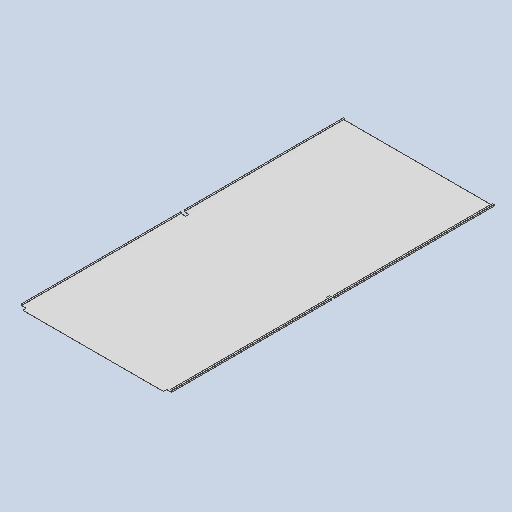
# Autodesk Inventor part: MSC 802 sheet gills
Saved by Autodesk Inventor 2025 (Build 290162010, 162A)
## iProperties
Created: 2024-06-15
Part Number: MSC 802 sheet gills
Material: Stainless Steel
Document SubType Name: Sheet Metal
Designer: pokla
Density: 8 g/cm^3
Sheet Metal Rule: Default_mm
Appearance: Default
Stock Number: МОО 802 лист жабра
Mass: 7522.03 g
Surface Area: 37640.3 cm^2
Volume: 940.254 cm^3
Flat Pattern Width: 95.1524 cm
Flat Pattern Length: 198 cm
Flat Pattern Area: 18840.2 cm^2
Sheet Metal Width: 951,524 mm
Sheet Metal Length: 1980,000 mm
Sheet Metal Area: 1884017,309 mm^2
Author: pokla
Autodesk Inventor part; units mm, degrees
ref_plane "YZ Plane" through (0, 0, 0) normal (1, 0, 0) x (0, 1, 0)
ref_plane "XZ Plane" through (0, 0, 0) normal (0, 1, 0) x (-1, 0, 0)
ref_plane "XY Plane" through (0, 0, 0) normal (0, 0, 1) x (1, 0, 0)
sketch "Sketch6" plane through (0, 0, 0) normal (0, 1, 0) x (-1, 0, 0)
  line L0 (457.5, -990) -> (-457.5, -990)
  line L1 (-457.5, -990) -> (-457.5, 990)
  line L2 (-457.5, 990) -> (457.5, 990)
  line L3 (457.5, 990) -> (457.5, -990)
  line L4 (457.5, -990) -> (-457.5, 990) construction
  line L5 (-457.5, -990) -> (457.5, 990) construction
  point P0 (0, 0)
  dimension "d52" = 915
  dimension "d53" = 1980
  measures "d52" distance of L1.end L2.end
  measures "d53" distance of L0.end L1.end
extrude "Plate2" add sketch "Sketch6" along normal blind 0.5
sketch "Sketch10" plane through (-457, 0, 990) normal (-1, 0, 0) x (0, -1, 0)
  line L0 (0, -1980) -> (0, 0)
  line L1 (0, 0) -> (-10, 0)
  line L2 (-10, 0) -> (-10, -1980)
  line L3 (-10, -1980) -> (0, -1980)
  constraints: 6 end point, 1 horizontal, 1 perpendicular, 1 vertical
edge flange "Flange1" height 10 angle 90 thickness 0.5 bend radius 0.5 thickness toward (-1, 0, 0) relief straight relief width 0.5 relief depth 0.25 corner gap 0.5 corner form 0 edges at (-457.5, 0.5, 0) (457.5, 0.5, 0) wall of the first edge with corners at (-457, 0, -990) (-457, 0, 990) (-457, 10, 990) (-457, 10, -990)
bend "Bend2"
corner "Corner2"
sketch "Sketch11" plane through (457.5, 9.5, -990) normal (0, 1, 0) x (-1, 0, 0)
  line L0 (0, 1980) -> (0, 0)
  line L1 (0, 0) -> (10, 0)
  line L2 (10, 0) -> (10, 1980)
  line L3 (10, 1980) -> (0, 1980)
  constraints: 6 end point, 1 horizontal, 1 perpendicular, 1 vertical
edge flange "Flange2" height 10 angle 90 thickness 0.5 bend radius 0.5 thickness toward (0, 1, 0) relief straight relief width 0.5 relief depth 0.25 corner gap 0.5 corner form 0 edges at (457, 10, 0) (-457, 10, 0) wall of the first edge with corners at (457.5, 9.5, 990) (457.5, 9.5, -990) (447.5, 9.5, -990) (447.5, 9.5, 990)
bend "Bend3"
corner "Corner3"
sketch "Sketch12" plane through (0, 0, 0) normal (0, -1, 0) x (1, 0, 0)
  line L0 (457.5, -990) -> (457.5, 990) projected
  line L1 (457.5, 990) -> (457.5, -990) projected
  line L2 (-457.5, 990) -> (-427.5, 990)
  line L3 (-427.5, 990) -> (-427.5, 970)
  line L4 (-427.5, 970) -> (-457.5, 970)
  line L5 (-457.5, 970) -> (-457.5, 990)
  line L6 (-457.5, 0) -> (-427.5, 0)
  line L7 (-427.5, 0) -> (-427.5, -20)
  line L8 (-427.5, -20) -> (-457.5, -20)
  line L9 (-457.5, -20) -> (-457.5, 0)
  line L10 (457.5, 0) -> (427.5, 0)
  line L11 (427.5, 0) -> (427.5, -20)
  line L12 (427.5, -20) -> (457.5, -20)
  line L13 (457.5, -20) -> (457.5, 0)
  line L14 (456.5, -990) -> (456.5, 990) construction
  line L15 (457.5, 990) -> (427.5, 990)
  line L16 (427.5, 990) -> (427.5, 970)
  line L17 (427.5, 970) -> (457.5, 970)
  line L18 (457.5, 970) -> (457.5, 990)
  line L19 (-456.5, 990) -> (456.5, 990) projected
  line L20 (-457.5, -990) -> (-457.5, 990) projected
  point P0 (0, 0)
  point P1 (457.5, -20)
  point P2 (457.5, 0)
  point P3 (457.5, 970)
  dimension "d96" = 20
  dimension "d97" = 30
  dimension "d109" = 990
  dimension "d110" = 30
  constraints: 32 end point, 8 parallel, 4 collinear, 4 horizontal, 4 perpendicular, 3 equal length, 1 midpoint
  measures "d96" distance of L2.end L3.end
  measures "d97" distance of L2.start L2.end
  measures "d109" distance between parallel lines of L6 L2
  measures "d110" distance of L16.end L17.end
extrude "Extrusion3" cut sketch "Sketch12" against normal through all
fillet "Corner Round1" radius 4 16 edges at (-427.5, 0.25, 990) (-427.5, 0.25, 970) (-447.5, 9.75, 970) (427.5, 0.25, 990) (447.5, 9.75, 970) (427.5, 0.25, 970) (447.5, 9.75, 0) (447.5, 9.75, -20) (427.5, 0.25, -20) (427.5, 0.25, 0) (447.5, 9.75, -990) (-447.5, 9.75, -990) (-447.5, 9.75, 0) (-427.5, 0.25, 0) (-427.5, 0.25, -20) (-447.5, 9.75, -20)
equation "\"d52\" = ЖАБРЫ_базовая_ширина"
equation "\"d53\" = ЖАБРЫ_базовая_длина_дл_лист"
equation "\"d110\" = d97"
equation "\"d54\" = Thickness"
equation "\"d74\" = BendReliefWidth"
equation "\"d75\" = BendReliefDepth"
equation "\"d76\" = MinimumRemnant"
equation "\"d77\" = TransitionRadius"
equation "\"d80\" = BendRadius"
equation "\"d81\" = CornerReliefSize"
equation "\"d82\" = GapSize"
equation "\"d83\" = JacobiRadiusSize"
equation "\"d84\" = BendReliefWidth"
equation "\"d85\" = BendReliefDepth"
equation "\"d86\" = MinimumRemnant"
equation "\"d87\" = TransitionRadius"
equation "\"d90\" = BendRadius"
equation "\"d91\" = CornerReliefSize"
equation "\"d92\" = GapSize"
equation "\"d93\" = JacobiRadiusSize"
equation "\"BendRadius\" = Thickness"
equation "\"BendReliefWidth\" = Thickness"
equation "\"BendReliefDepth\" = 0.5 * Thickness"
equation "\"CornerReliefSize\" = 4 * Thickness"
equation "\"MinimumRemnant\" = 2 * Thickness"
equation "\"TransitionRadius\" = BendRadius"
equation "\"JacobiRadiusSize\" = BendRadius"
equation "\"GapSize\" = Thickness"
equation "\"ЖАБРЫ_базовая_ширина\" = 915"
equation "\"ЖАБРЫ_базовая_длина_дл_лист\" = 1980"
equation "\"Thickness\" = 0.5"
body "Solid2"
